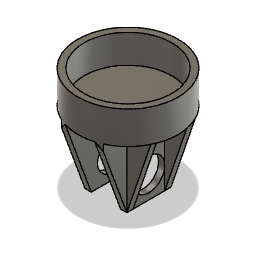
BearingWheelMount (Autodesk Fusion 360 design; units mm, degrees)
Autodesk Fusion 360 part; units mm, degrees
sketch "Sketch1" plane through (0, 0, 0) normal (0, 1, 0) x (1, 0, 0)
  circle A0 centre (0, 0) radius 11.22
  circle A1 centre (0, 0) radius 12.82
  dimension "d1" = 22.44
  dimension "d2" = 25.64
  constraint coincident A0.centre A1.centre
  measures "d1" diameter of A0
  measures "d2" diameter of A1
extrude "Extrude1" add sketch "Sketch1" along normal blind 1 contours A0 | A1
extrude "Extrude2" add sketch "Sketch1" along normal blind 8.3
sketch "Sketch2" plane through (0, 0, 0) normal (0, 0, 1) x (1, 0, 0)
  line L0 (3.75, -18.22) -> (3.75, 0)
  line L1 (-3.75, 0) -> (-3.75, -18.22)
  line L2 (11.22, 0) -> (-11.22, 0)
  line L3 (-3.75, -18.22) -> (-5.35, -18.22)
  line L4 (-5.35, -18.22) -> (-5.35, 0)
  line L5 (3.75, -18.22) -> (5.35, -18.22)
  line L6 (5.35, -18.22) -> (5.35, 0)
  dimension "d7" = 3.75
  dimension "d8" = 7.5
  dimension "d9" = 1.6
  dimension "d10" = 18.22
  constraint vertical L0
  constraint vertical L1
  constraint coincident L0.end L2
  constraint coincident L1.start L2
  constraint horizontal L0.start L1.end
  constraint perpendicular L1 L3
  constraint coincident L2 L4.end
  constraint perpendicular L2 L4
  constraint perpendicular L0 L5
  constraint coincident L2 L6.end
  constraint perpendicular L2 L6
  constraint equal L3 L5
  measures "d7" distance of L0 origin
  measures "d8" distance of L0 L1
  measures "d9" distance of L1.end L3.end
  measures "d10" distance of L3.end L4.end
extrude "Extrude4" add sketch "Sketch2" along normal blind 5.65
extrude "Extrude5" add sketch "Sketch2" against normal blind 5.65
sketch "Sketch4" plane through (3.75, 0, 0) normal (-1, 0, 0) x (0, 0, 1)
  line L0 (-5.65, -18.22) -> (5.65, -18.22)
  line L1 (5.65, -18.22) -> (5.65, 0)
  line L2 (5.65, 0) -> (-5.65, 0)
  circle A0 centre (0, -12.57) radius 4.05
  line L3 (-4.05, -12.57) -> (-5.65, -12.57) construction
  line L4 (4.05, -12.57) -> (5.65, -12.57) construction
  line L5 (0, -16.62) -> (0, -18.22) construction
  line L6 (-5.65, 0) -> (-5.65, -18.22)
  dimension "d23" = 8.1
  constraint coincident A0 L3.start
  constraint coincident A0 L4.start
  constraint coincident L1 L4.end
  constraint horizontal L4
  constraint collinear L3 L4
  constraint equal L3 L4
  constraint coincident A0 L5.start
  constraint midpoint L0 L5.end
  constraint perpendicular L0 L5
  constraint equal L3 L5
  constraint collinear A0.centre L3.end L4.end
  constraint coincident L3.end L6
  measures "d23" diameter of A0
sketch "Sketch3" plane through (-4.45, -11.11, -5.65) normal (0, 0, -1) x (1, 0, 0)
  line L0 (9.8, 7.11) -> (15.9578, -11.11)
  circle A0 through (-8.37, -11.11, -5.65) (10.86, -11.11, 5.4524) (10.86, -11.11, -16.7524)
  line L1 (9.8, -11.11) -> (9.8, 7.11)
  line L2 (9.8, -11.11) -> (15.9578, -11.11) construction
  line L3 (15.9578, -11.11) -> (9.8, -11.11)
  line L4 (-0.8, -11.11) -> (-7.0578, -11.11)
  line L5 (-0.9, 7.11) -> (-0.9, -11.11)
  line L6 (-7.0578, -11.11) -> (-0.9, 7.11)
  point P0 (9.8, 7.11)
  point P1 (-0.9, -11.11)
  constraint coincident L1.start L2.start
  constraint perpendicular L1 L2
  constraint coincident L0.end L2
  constraint coincident L0.end L2.end
  constraint horizontal L4
  constraint collinear L3 L4
  constraint coincident L5.start L6.end
  constraint coincident P0 L0.start
extrude "Extrude6" add sketch "Sketch3" against normal blind 1.6
extrude "Extrude7" cut sketch "Sketch4" along normal through all contours A0
extrude "Extrude8" cut sketch "Sketch4" against normal blind 8 contours A0
mirror "Mirror1" about plane through (0, 0, 0) normal (0, 0, 1) of "Extrude6"
sketch "Sketch5" plane through (-3.75, 0, 0) normal (1, 0, 0) x (0, 0, -1)
  line L0 (-5.65, 0) -> (-5.65, -18.22)
  line L1 (-5.65, -18.22) -> (5.65, -18.22)
  line L2 (5.65, -18.22) -> (5.65, 0)
  line L3 (5.65, 0) -> (-5.65, 0)
  circle A0 centre (0, -12.57) radius 4.05
  arc A1 through (5.65, 0, -7.7578) (12.82, 0, 3.75) (5.65, 0, 15.2578)
  line L4 (5.65, -18.22) -> (12.2593, 0)
  line L5 (-5.65, 0) -> (5.65, 0)
  line L6 (12.2593, 0) -> (5.65, 0)
  arc A2 through (-5.65, 0, 15.2578) (-12.82, 0, 3.75) (-5.65, 0, -7.7578)
  line L7 (-5.65, 0) -> (-12.2593, 0)
  line L8 (-12.2593, 0) -> (-5.65, -18.22)
  constraint coincident L1.end L2.start
  constraint collinear L0.start L2.end L4.end
  constraint coincident L2.end L3.start
  constraint coincident L0.start L3.end
  constraint coincident L0.end L1.start
  constraint collinear L3 L7
extrude "Extrude9" add sketch "Sketch5" against normal blind 1.6 contours L0 L7 L8 | L2 L4 L6
mirror "Mirror2" about plane through (0, 0, 0) normal (1, 0, 0) of "Extrude9"
sketch "Sketch6" plane through (0, 0, 0) normal (0, -1, 0) x (1, 0, 0)
  line L0 (3.75, -12.2593) -> (3.75, 12.2593)
  arc A0 (3.75, 12.2593) -> (-3.75, 12.2593) centre (0, 0) ccw
  line L1 (-3.75, 12.2593) -> (-3.75, -12.2593)
  arc A1 (-3.75, -12.2593) -> (3.75, -12.2593) centre (0, 0) ccw
  circle A2 centre (0, 0) radius 12.82
  circle A3 centre (0, 0) radius 15
  dimension "d35" = 30
  constraint concentric A0 A2
  constraint concentric A2 A3
  constraint tangent A1 A2
  measures "d35" diameter of A3
extrude "Extrude10" cut sketch "Sketch6" along normal blind 9 contours L0 A0 L1 A1 A2 | A3
equation "d2 = d1 + 3.2 mm"
equation "d7 = d8 / 2"
equation "d15 = -( 11.30 / 2 ) * 1 mm"
equation "d19 = ( 11.30 / 2 ) * 1 mm"
